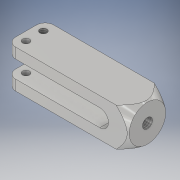
# Autodesk Inventor part: middle handle piece (hard) (1)
Saved by Autodesk Inventor 2017 (Build 210142000, 142)
## iProperties
Created: 2017-04-14
Part Number: middle handle piece (hard) (1)
Material: Aluminum 6061
Document SubType Name: Modeling
Designer: 193515
Density: 2.7 g/cm^3
Appearance: Aluminum - Dark
Author: 193515
Autodesk Inventor part; units mm, degrees
ref_plane "YZ Plane" through (0, 0, 0) normal (1, 0, 0) x (0, 1, 0)
ref_plane "XZ Plane" through (0, 0, 0) normal (0, 1, 0) x (-1, 0, 0)
sketch "Sketch1" plane through (0, 0, 0) normal (0, 0, 1) x (1, 0, 0)
  line L0 (0, 0) -> (111.125, 0)
  line L1 (111.125, 0) -> (111.125, 34.925)
  line L2 (111.125, 34.925) -> (0, 34.925)
  arc A0 (85.0138, 9.525) -> (85.0138, 25.4) centre (85.0138, 17.4625) ccw
  line L3 (85.0138, 25.4) -> (0, 25.4)
  line L4 (0, 9.525) -> (85.0138, 9.525)
  line L5 (85.0138, 9.525) -> (85.0138, 25.4)
  line L6 (0, 34.925) -> (0, 25.4)
  line L7 (0, 9.525) -> (0, 0)
  dimension "d0" = 34.925
  dimension "d2" = 15.875
  dimension "d3" = 85.0138
  dimension "d4" = 111.125
  constraints: 16 end point, 4 parallel, 2 horizontal, 2 point on circle, 1 centre point, 1 perpendicular, 1 vertical alignment
  measures "d0" distance of L2.end L0.start
  measures "d2" diameter of A0
  measures "d3" distance between parallel lines of L5 L7
  measures "d4" distance of L0.start L0.end
extrude "Extrusion1" add sketch "Sketch1" along normal blind 34.925 contours L7 L4 A0 L3 L6 L2 L1 L0
sketch "Sketch2" plane through (111.125, 0, 0) normal (1, 0, 0) x (0, 0, -1)
  point P0 (0, 0)
  point P1 (-17.4625, 17.4752)
hole "Hole1" at (111.125, 17.4752, 17.4625) direction (-1, 0, 0) diameter 9.144 end through all thread size "7/16-14 UNC" class "2B" standard "ANSI Unified Screw Threads"
ref_plane "Work Plane1" through (111.125, 34.925, 0) normal (0, 0.7071, 0.7071) x (-1, 0, 0)
sketch "Sketch3" plane through (111.125, 34.925, 0) normal (0, 0.7071, 0.7071) x (-1, 0, 0)
  line L0 (0, 0) -> (111.125, 0) projected
  line L1 (111.125, 0) -> (111.125, 24.6957) projected
  line L2 (0, 24.6957) -> (111.125, 24.6957) projected
  line L3 (0, 0) -> (0, 24.6957) projected
  line L4 (0, 0) -> (0, 24.6957) projected
  line L5 (0, 8.027) -> (11.1125, 0)
  line L6 (11.1125, 0) -> (0, 0)
  line L7 (0, 8.027) -> (0, 0)
  dimension "d14" = 11.1125
  dimension "d15" = 16.6687
  constraints: 6 end point, 2 collinear, 2 point on line
  measures "d14" distance from line of L5.end L3
  measures "d15" distance of L5.start L2.start
revolve "Revolution1" cut sketch "Sketch3" angle 360 about axis through (111.125, 17.4625, 17.4625) along (-1, 0, 0) contours L3 L5 L0
fillet "Fillet1" radius 7.9375 4 edges at (0, 30.1625, 0) (0, 4.7625, 0) (0, 4.7625, 34.925) (0, 30.1625, 34.925)
sketch "Sketch4" plane through (7.9375, 0, 0) normal (0, -1, 0) x (1, 0, 0)
  point P0 (-7.9375, 0)
  point P1 (0, 9.525)
  point P2 (0, 25.4)
sketch "Sketch5" plane through (7.9375, 34.925, 0) normal (0, 1, 0) x (1, 0, 0)
  line L0 (92.075, -34.925) -> (0, -34.925) projected
  line L1 (92.075, 0) -> (0, 0) projected
  point P0 (-7.9375, 0)
  dimension "d18" = 34.925
  measures "d18" distance between parallel lines of L0 L1
sketch "Sketch6" plane through (7.9375, 34.925, 0) normal (0, 1, 0) x (1, 0, 0)
  point P0 (-7.9375, 0)
  point P1 (0, -9.525)
  point P2 (0, -25.4)
hole "Hole2" at (7.9375, 34.925, 9.525) direction (0, -1, 0) diameter 6.4008 depth 83.2612 tip angle 118 thread size "5/16-18 UNC" class "2B" standard "ANSI Unified Screw Threads"
thread "Thread1" size "5/16-18 UNC" class "2B" standard "ANSI Unified Screw Threads" full length
sketch "Sketch7" plane through (7.9375, 34.925, 0) normal (0, 1, 0) x (1, 0, 0)
  point P0 (-7.9375, 0)
  point P1 (0, -25.4)
hole "Hole3" at (7.9375, 34.925, 25.4) direction (0, -1, 0) diameter 6.35 end through all
body "Solid1"
